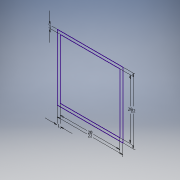
# Autodesk Inventor part: brazo
Saved by Autodesk Inventor 2018 (Build 220112000, 112)
## iProperties
Created: 2021-07-10
Part Number: brazo
Material: Genérico
Document SubType Name: Modeling
Designer: GABRIEL
Density: 1 g/cm^3
Appearance: Valor por defecto
Author: GABRIEL
Autodesk Inventor part; units mm, degrees
ref_plane "YZ Plane" through (0, 0, 0) normal (1, 0, 0) x (0, 1, 0)
ref_plane "XZ Plane" through (0, 0, 0) normal (0, 1, 0) x (-1, 0, 0)
ref_plane "XY Plane" through (0, 0, 0) normal (0, 0, 1) x (1, 0, 0)
sketch "Boceto1" plane through (0, 0, 0) normal (0, 1, 0) x (-1, 0, 0)
  line L0 (0, 0) -> (-10, 0)
  line L1 (-10, 0) -> (-10, -10)
  line L2 (-10, -10) -> (0, -10)
  line L3 (0, -10) -> (0, 0)
  line L4 (1, 1) -> (-11, 1)
  line L5 (-11, 1) -> (-11, -11)
  line L6 (-11, -11) -> (1, -11)
  line L7 (1, -11) -> (1, 1)
  dimension "d0" = 10
  dimension "d2" = 12
  dimension "d4" = 1
  dimension "d5" = 1
  constraints: 16 end point, 4 parallel, 4 perpendicular, 2 horizontal
  measures "d0" distance of L2.end L1.end
  measures "d2" distance of L6.end L5.end
  measures "d4" distance between parallel lines of L4 L0
  measures "d5" distance between parallel lines of L3 L7
extrude "Extrusión1" add sketch "Boceto1" along normal blind 160
sketch "Boceto2" plane through (-1, 0, -11) normal (-1, 0, 0) x (0, 0, 1)
  circle A0 centre (6, 10) radius 4
  circle A1 centre (6, 30.28) radius 4
  line L0 (0, 0) -> (12, 0) projected
  line L1 (0, 0) -> (0, 160) projected
  circle A2 centre (6, 150) radius 4
  line L2 (0, 160) -> (12, 160) projected
  dimension "d8" = 8
  dimension "d9" = 8
  dimension "d11" = 20.28
  dimension "d14" = 10
  dimension "d15" = 6
  dimension "d16" = 6
  dimension "d17" = 8
  dimension "d18" = 6
  dimension "d19" = 10
  constraints: 3 centre point
  measures "d8" diameter of A0
  measures "d9" diameter of A1
  measures "d11" distance of A1.centre A0.centre
  measures "d14" distance from line of L0 A0.centre
  measures "d15" distance from line of L1 A0.centre
  measures "d16" distance from line of L1 A1.centre
  measures "d17" diameter of A2
  measures "d18" distance from line of L1 A2.centre
  measures "d19" distance from line of L2 A2.centre
extrude "Extrusión2" cut sketch "Boceto2" against normal blind 20
